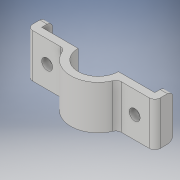
# Autodesk Inventor part: SólidoA
Saved by Autodesk Inventor 2018 (Build 220112000, 112)
## iProperties
Created: 2017-10-07
Part Number: SólidoA
Material: Generic
Document SubType Name: Modeling
Designer: Soichi
Density: 1 g/cm^3
Appearance: Default
Author: Soichi
Autodesk Inventor part; units mm, degrees
ref_plane "YZ Plane" through (0, 0, 0) normal (1, 0, 0) x (0, 1, 0)
ref_plane "XZ Plane" through (0, 0, 0) normal (0, 1, 0) x (-1, 0, 0)
ref_plane "XY Plane" through (0, 0, 0) normal (0, 0, 1) x (1, 0, 0)
sketch "Sketch1" plane through (0, 0, 0) normal (0, 1, 0) x (-1, 0, 0)
  line L0 (98.425, 0) -> (98.425, -19.05)
  line L1 (98.425, -19.05) -> (111.125, -19.05)
  line L2 (111.125, -19.05) -> (111.125, 12.7)
  line L3 (111.125, 12.7) -> (46.0322, 12.7)
  arc A0 (35.052, 0) -> (0, 35.052) centre (0, 0) ccw
  line L4 (0, 0) -> (35.052, 0) construction
  line L5 (0, 0) -> (35.052, 0) construction
  line L6 (0, 0) -> (0, 47.752) construction
  arc A1 (46.0322, 12.7) -> (0, 47.752) centre (0, 0) ccw
  line L7 (35.052, 0) -> (98.425, 0)
  line L8 (-98.425, 0) -> (-98.425, -19.05)
  line L9 (-98.425, -19.05) -> (-111.125, -19.05)
  line L10 (-111.125, -19.05) -> (-111.125, 12.7)
  line L11 (-111.125, 12.7) -> (-46.0322, 12.7)
  arc A2 (0, 35.052) -> (-35.052, 0) centre (0, 0) ccw
  arc A3 (0, 47.752) -> (-46.0322, 12.7) centre (0, 0) ccw
  line L12 (-35.052, 0) -> (-98.425, 0)
  arc A4 (35.052, 0) -> (-35.052, 0) centre (0, 0) ccw
  arc A5 (46.0322, 12.7) -> (-46.0322, 12.7) centre (0, 0) ccw
  line L13 (35.052, 0) -> (98.425, 0)
  line L14 (98.425, 0) -> (98.425, -19.05)
  line L15 (111.125, -19.05) -> (111.125, 12.7)
  line L16 (46.0322, 12.7) -> (111.125, 12.7)
  line L17 (-46.0322, 12.7) -> (-111.125, 12.7)
  line L18 (-111.125, -19.05) -> (-111.125, 12.7)
  line L19 (-98.425, -19.05) -> (-111.125, -19.05)
  line L20 (-98.425, 0) -> (-35.052, 0)
  line L21 (-98.425, 0) -> (-35.052, 0)
  dimension "d7" = 12.7
  dimension "d9" = 35.052
  dimension "d10" = 0
  dimension "d11" = 90
  dimension "d12" = 12.7
  dimension "d13" = 31.75
  dimension "d14" = 12.7
  dimension "d30" = 98.425
  constraints: 44 end point, 12 point on circle, 9 collinear, 7 symmetric about line, 6 centre point, 3 coincident, 3 perpendicular, 2 point on line, 1 horizontal, 2 other
  measures "d7" distance of L0.end L1.end
  measures "d9" radius of A0
  measures "d10" distance between parallel lines of L4 L5
  measures "d11" angle of L4 L6
  measures "d12" radial gap between concentric circles of A0 A1
  measures "d13" distance between parallel lines of L3 L1
  measures "d14" distance between parallel lines of L3 L7
  measures "d30" distance from line of L0 point (0, 0)
extrude "Extrusion1" add sketch "Sketch1" along normal blind 76.2
fillet "Fillet1" radius 9.652 8 edges at (111.125, 38.1, 12.7) (46.0322, 38.1, 12.7) (104.775, 76.2, -19.05) (104.775, 0, -19.05) (-46.0322, 38.1, 12.7) (-111.125, 38.1, 12.7) (-104.775, 0, -19.05) (-104.775, 76.2, -19.05)
sketch "Sketch2" plane through (52.8735, 0, 12.7) normal (0, 0, 1) x (1, 0, 0)
  line L0 (-52.8735, 0) -> (-52.8735, 38.1) construction
  line L1 (-52.8735, 38.1) -> (-129.0735, 38.1) construction
  line L2 (-52.8735, 38.1) -> (23.3265, 38.1) construction
  dimension "d20" = 38.1
  dimension "d21" = 76.2
  dimension "d22" = 76.2
  constraints: 6 end point, 2 coincident, 1 horizontal, 1 perpendicular, 1 vertical
  measures "d20" distance of L0.start L0.end
  measures "d21" distance of L0.end L1.end
  measures "d22" distance of L0.end L2.end
hole "Hole1" at (-76.2, 38.1, 12.7) at (76.2, 38.1, 12.7) direction (0, 0, -1) diameter 19.05 end through all
body "Solid1"
